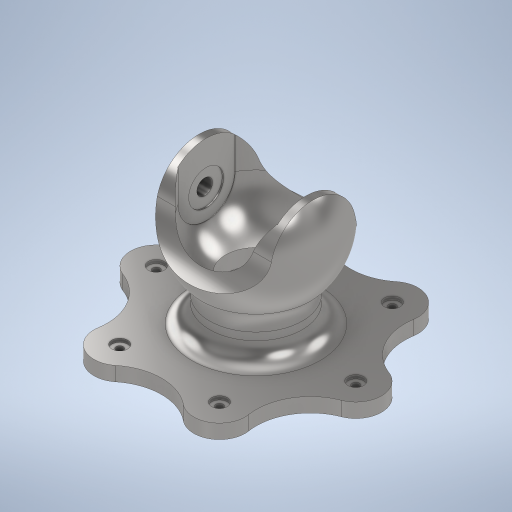
# Autodesk Inventor part: giunto_sferico
Saved by Autodesk Inventor 2023 (Build 270158000, 158)
## iProperties
Created: 2023-07-04
Part Number: giunto_sferico
Material: Acciaio inossidabile
Document SubType Name: Modeling
Designer: nicol
Density: 8 g/cm^3
Appearance: Semilucidato
Author: nicol
Autodesk Inventor part; units mm, degrees
ref_plane "YZ Plane" through (0, 0, 0) normal (1, 0, 0) x (0, 1, 0)
ref_plane "XZ Plane" through (0, 0, 0) normal (0, 1, 0) x (-1, 0, 0)
ref_plane "XY Plane" through (0, 0, 0) normal (0, 0, 1) x (1, 0, 0)
sketch "Schizzo1" plane through (0, 0, 0) normal (0, 1, 0) x (-1, 0, 0)
  circle A0 centre (0, 0) radius 140 construction
  arc A1 (-135.371429, 35.701209) -> (-135.371429, -35.701209) centre (-140, 0) ccw
  arc A2 (-98.603868, -99.384492) -> (-36.76756, -135.085701) centre (-70, -121.243557) ccw
  arc A3 (36.76756, -135.085701) -> (98.603868, -99.384492) centre (70, -121.243557) ccw
  arc A4 (135.371429, -35.701209) -> (135.371429, 35.701209) centre (140, 0) ccw
  arc A5 (98.603868, 99.384492) -> (36.76756, 135.085701) centre (70, 121.243557) ccw
  arc A6 (-36.76756, 135.085701) -> (-98.603868, 99.384492) centre (-70, 121.243557) ccw
  arc A7 (47.5, -149.346048) -> (-47.5, -149.346048) centre (0, -208.673529) ccw
  arc A8 (153.087471, -33.536817) -> (105.587471, -115.80923) centre (180.716577, -104.336764) ccw
  arc A9 (105.587471, 115.80923) -> (153.087471, 33.536817) centre (180.716577, 104.336764) ccw
  arc A10 (-47.5, 149.346048) -> (47.5, 149.346048) centre (0, 208.673529) ccw
  arc A11 (-153.087471, 33.536817) -> (-105.587471, 115.80923) centre (-180.716577, 104.336764) ccw
  arc A12 (-105.587471, -115.80923) -> (-153.087471, -33.536817) centre (-180.716577, -104.336764) ccw
  point P0 (-153.087471, -33.536817)
  point P1 (105.587471, -115.80923)
  point P2 (153.087471, -33.536817)
  point P3 (153.087471, 33.536817)
  point P4 (105.587471, 115.80923)
  point P5 (47.5, 149.346048)
  point P6 (-47.5, 149.346048)
  point P7 (-105.587471, 115.80923)
  point P8 (-153.087471, 33.536817)
  dimension "d0" = 280
  dimension "d1" = 72
  dimension "d4" = 360
  dimension "d7" = 152
  dimension "d10" = 360
  constraints: 29 point on circle, 13 centre point, 8 coincident, 2 tangent, 60 other
  measures "d0" diameter of A0
  measures "d1" diameter of A1
  measures "d7" diameter of A7
extrude "Estrusione1" add sketch "Schizzo1" along normal blind 20
sketch "Schizzo2" plane through (0, 20, 0) normal (0, 1, 0) x (1, 0, 0)
  arc A0 (47.5, -149.346048) -> (105.587471, -115.80923) centre (70, -121.243557) ccw
  point P0 (0, 0)
  constraints: 1 coincident
hole "Foro1" at (70, 20, 121.243557) direction (0, -1, 0) diameter 10 end through all counterbore diameter 22 counterbore depth 5
sketch "Schizzo3" plane through (0, 0, 0) normal (0, -1, 0) x (1, 0, 0)
  arc A0 (105.587471, 115.80923) -> (47.5, 149.346048) centre (70, 121.243557) ccw
  point P0 (0, 0)
  constraints: 1 coincident
hole "Foro2" at (70, 0, 121.243557) direction (0, 1, 0) diameter 35 depth 2
pattern_circular "Serie circolare1" count 6 over 360 about axis through (0, -10, 0) along (0, 1, 0) of "Foro1", "Foro2"
sketch "Schizzo4" plane through (0, 0, 0) normal (0, 0, 1) x (1, 0, 0)
  arc A0 (65, 74.006579) -> (0, 250) centre (0, 150) ccw
  line L0 (176, 0) -> (153.087471, 0)
  line L1 (0, 250) -> (0, 50)
  line L2 (65, 74.006579) -> (65, 20)
  line L3 (106, 20) -> (47.5, 20)
  line L4 (106, 20) -> (47.5, 20)
  line L5 (-47.5, 0) -> (47.5, 0)
  line L6 (0, 50) -> (0, 20)
  line L7 (-47.5, 20) -> (47.5, 20)
  line L8 (0, 20) -> (65, 20)
  point P0 (0, 0)
  point P1 (105.587471, 20)
  point P2 (0, 0)
  dimension "d32" = 200
  dimension "d33" = 150
  dimension "d34" = 65
  constraints: 8 end point, 2 midpoint, 2 point on circle, 1 centre point, 1 collinear, 1 perpendicular, 1 point on line, 1 vertical
  measures "d32" diameter of A0
  measures "d33" distance from line of A0.centre L0
  measures "d34" distance from line of point (0, 0) L2
revolve "Rivoluzione1" add sketch "Schizzo4" angle 360 about axis through (0, 250, 0) along (0, -1, 0)
fillet "Raccordo1" radius 25 1 edges at (-65, 20, 0)
fillet "Raccordo2" radius 45 1 edges at (-65, 74.0066, 0)
sketch "Schizzo5" plane through (0, 0, 0) normal (1, 0, 0) x (0, 1, 0)
  arc A0 (84.846746, -75.862069) -> (84.846746, 75.862069) centre (150, 0) ccw
  arc A1 (163.714286, -58.411629) -> (163.714286, 58.411629) centre (150, 0) ccw
  arc A2 (114.43261, 93.461012) -> (163.714286, 58.411629) centre (182, 136.2938) ccw
  arc A3 (163.714286, -58.411629) -> (114.43261, -93.461012) centre (182, -136.2938) ccw
  point P0 (0, 0)
  point P1 (114.43261, -93.461012)
  dimension "d38" = 120
  dimension "d39" = 160
  dimension "d40" = 182
  constraints: 7 point on circle, 3 centre point, 1 coincident, 1 tangent
  measures "d38" diameter of A1
  measures "d39" diameter of A2
  measures "d40" horizontal distance of A2.centre point (0, 0)
extrude "Estrusione2" cut sketch "Schizzo5" along normal through all both and the other way through all
sketch "Schizzo6" plane through (0, 0, 0) normal (0, -1, 0) x (1, 0, 0)
  circle A0 centre (0, 0) radius 65 projected
  circle A1 centre (0, 0) radius 76
  circle A2 centre (0, 0) radius 60
  dimension "d43" = 152
  dimension "d44" = 120
  constraints: 2 centre point, 2 coincident
  measures "d43" diameter of A1
  measures "d44" diameter of A2
extrude "Estrusione3" add sketch "Schizzo6" along normal blind 6 contours A0 | A1
sketch "Schizzo7" plane through (0, 0, 0) normal (0, 0, 1) x (1, 0, 0)
  point P0 (0, 0)
sketch "Schizzo8" plane through (0, 0, 0) normal (0, 0, 1) x (1, 0, 0)
  arc A0 (-80, 210) -> (80, 210) centre (0, 150) ccw
  arc A1 (0, 230) -> (-42.5, 82.222791) centre (0, 150) ccw
  line L0 (-42.5, 82.222791) -> (-42.5, 40)
  line L1 (-42.5, 40) -> (-32, 40)
  line L2 (-32, 40) -> (-32, -34.251935)
  line L3 (-32, -34.251935) -> (0, -34.251935)
  line L4 (0, -34.251935) -> (0, 230)
  line L5 (-60, 0) -> (60, 0)
  point P0 (0, 0)
  point P1 (0, 97.874032)
  point P2 (-37.25, 40)
  point P3 (-42.5, 59.480665)
  point P4 (0, 50)
  dimension "d47" = 160
  dimension "d48" = 42.5
  dimension "d49" = 32
  dimension "d50" = 40
  constraints: 10 end point, 3 perpendicular, 2 midpoint, 2 point on circle, 2 vertical, 1 centre point, 1 coincident, 1 vertical alignment
  measures "d47" diameter of A1
  measures "d48" distance between parallel lines of L4 L0
  measures "d49" distance between parallel lines of L4 L2
  measures "d50" distance from line of L5 point (-37.25, 40)
revolve "Rivoluzione2" cut sketch "Schizzo8" angle 360 about axis through (0, -34.251935, 0) along (0, 1, 0) contours L0 A1 L4 A0
sketch "Schizzo11" plane through (0, 0, 0) normal (1, 0, 0) x (0, 1, 0)
  line L0 (55.527782, -65) -> (55.527782, 65)
  arc A0 (163.714286, -58.411629) -> (163.714286, 58.411629) centre (150, 0) ccw
  arc A1 (150, 40) -> (150, -40) centre (150, 0) ccw
  line L1 (150, 40) -> (294.880914, 40)
  line L2 (294.880914, 40) -> (294.880914, -40)
  line L3 (294.880914, -40) -> (150, -40)
  point P0 (0, 0)
  dimension "d52" = 80
  constraints: 6 end point, 2 perpendicular, 2 point on circle, 1 centre point, 1 coincident, 1 horizontal, 1 tangent
  measures "d52" diameter of A1
extrude "Estrusione4" cut sketch "Schizzo11" along normal mid plane 140
ref_plane "Piano di lavoro1" through (0, 150, 0) normal (0, 1, 0) x (1, 0, 0)
sketch "Schizzo12" plane through (0, 150, 0) normal (0, 1, 0) x (1, 0, 0)
  arc A0 (49.340176, -62.972589) -> (-49.340176, -62.972589) centre (0, 0) ccw
  line L0 (-69.282032, 40) -> (-69.282032, -40)
  line L1 (69.282032, -40) -> (69.282032, 40)
  arc A1 (69.282032, 40) -> (-69.282032, 40) centre (0, 0) ccw
  arc A2 (-69.282032, -40) -> (69.282032, -40) centre (0, 0) ccw
  point P0 (-49.340176, -62.972589)
  constraints: 4 end point, 4 point on circle, 2 centre point, 1 coincident
extrude "Estrusione5" cut sketch "Schizzo12" along normal through all contours A2 A0 L0 L1
sketch "Schizzo13" plane through (-70, 0, 0) normal (1, 0, 0) x (0, 0, -1)
  circle A0 centre (0, 150) radius 38.729833
  point P0 (0, 0)
extrude "Estrusione6" add sketch "Schizzo13" against normal blind 20
mirror "Specchio1" about plane through (0, 0, 0) normal (1, 0, 0) of "Estrusione6"
sketch "Schizzo14" plane through (-70, 0, 0) normal (1, 0, 0) x (0, 0, -1)
  arc A0 (-40, 150) -> (40, 150) centre (0, 150) ccw projected
  point P0 (0, 0)
  constraints: 1 coincident
hole "Foro3" at (-70, 150, 0) direction (-1, 0, 0) diameter 22 depth 21 counterbore diameter 49 counterbore depth 2
